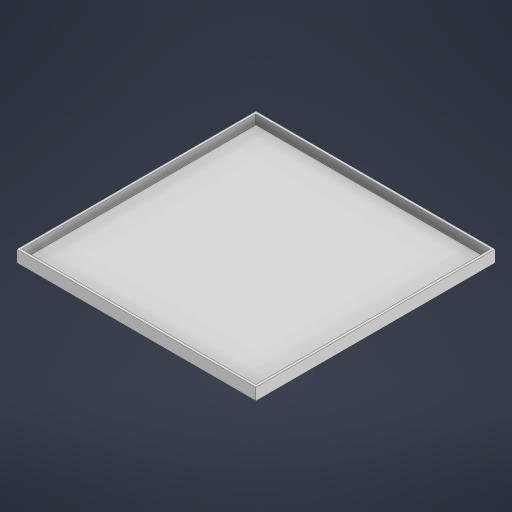
# Autodesk Inventor part: box
Saved by Autodesk Inventor 2024 (Build 280153000, 153)
## iProperties
Created: 2024-02-06
Part Number: box
Material: Všeobecné
Document SubType Name: Modeling
Designer: Simak
Density: 1 g/cm^3
Appearance: Výchozí
Author: Simak
Autodesk Inventor part; units mm, degrees
ref_plane "YZ Plane" through (0, 0, 0) normal (1, 0, 0) x (0, 1, 0)
ref_plane "XZ Plane" through (0, 0, 0) normal (0, 1, 0) x (-1, 0, 0)
ref_plane "XY Plane" through (0, 0, 0) normal (0, 0, 1) x (1, 0, 0)
sketch "Náčrt1" plane through (0, 0, 0) normal (0, 1, 0) x (-1, 0, 0)
  line L0 (49.75, -49.75) -> (-49.75, -49.75)
  line L1 (-49.75, -49.75) -> (-49.75, 49.75)
  line L2 (-49.75, 49.75) -> (49.75, 49.75)
  line L3 (49.75, 49.75) -> (49.75, -49.75)
  line L4 (49.75, -49.75) -> (0, 0) construction
  line L5 (0, 0) -> (-49.75, -49.75) construction
  line L6 (0, 0) -> (-49.75, 49.75) construction
  line L7 (50.75, -50.75) -> (-50.75, -50.75)
  line L8 (-50.75, -50.75) -> (-50.75, 50.75)
  line L9 (-50.75, 50.75) -> (50.75, 50.75)
  line L10 (50.75, 50.75) -> (50.75, -50.75)
  dimension "d0" = 99.5
  dimension "d3" = 1
  constraints: 22 end point, 8 equal length, 2 perpendicular, 1 horizontal, 3 other
  measures "d0" distance of L0.start L0.end
  measures "d3" distance between parallel lines of L3 L10
extrude "Vysunutí1" add sketch "Náčrt1" along normal blind 1 contours L0 L1 L2 L3
extrude "Vysunutí2" add sketch "Náčrt1" along normal blind 5
